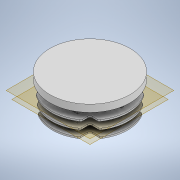
# Autodesk Inventor part: Plug
Saved by Autodesk Inventor 2020.2 (Build 242310000, 310)
## iProperties
Created: 2019-12-23
Part Number: Plug
Material: Générique
Document SubType Name: Modeling
Designer: damien
Density: 1 g/cm^3
Appearance: Par défaut
Author: damien
Autodesk Inventor part; units mm, degrees
ref_plane "YZ Plane" through (0, 0, 0) normal (1, 0, 0) x (0, 1, 0)
ref_plane "XZ Plane" through (0, 0, 0) normal (0, 1, 0) x (-1, 0, 0)
ref_plane "XY Plane" through (0, 0, 0) normal (0, 0, 1) x (1, 0, 0)
sketch "Esquisse1" plane through (0, 0, 0) normal (0, 1, 0) x (-1, 0, 0)
  line L0 (7.6, 13.55) -> (-7.6, 13.55)
  line L1 (-7.6, 13.55) -> (-7.6, 12.25)
  line L2 (-7.6, 12.25) -> (-0.65, 12.25)
  line L3 (-0.65, 12.25) -> (-0.65, 0.65)
  line L4 (-0.65, 0.65) -> (-15.5, 0.65)
  line L5 (-15.5, 0.65) -> (-15.5, -0.65)
  line L6 (-15.5, -0.65) -> (-0.65, -0.65)
  line L7 (-0.65, -0.65) -> (-0.65, -12.25)
  line L8 (-0.65, -12.25) -> (-7.6, -12.25)
  line L9 (-7.6, -12.25) -> (-7.6, -13.55)
  line L10 (-7.6, -13.55) -> (7.6, -13.55)
  line L11 (7.6, -13.55) -> (7.6, -12.25)
  line L12 (7.6, -12.25) -> (0.65, -12.25)
  line L13 (0.65, -12.25) -> (0.65, -0.65)
  line L14 (0.65, -0.65) -> (15.5, -0.65)
  line L15 (15.5, -0.65) -> (15.5, 0.65)
  line L16 (15.5, 0.65) -> (0.65, 0.65)
  line L17 (0.65, 0.65) -> (0.65, 12.25)
  line L18 (0.65, 12.25) -> (7.6, 12.25)
  line L19 (7.6, 12.25) -> (7.6, 13.55)
  line L20 (-0.65, 0.65) -> (0.65, -0.65) construction
  line L21 (0.65, 0.65) -> (-0.65, -0.65) construction
  point P0 (0, 0)
  point P1 (0, 0)
  dimension "d0" = 15.2
  dimension "d1" = 27.1
  dimension "d2" = 1.3
  dimension "d4" = 31
  dimension "d7" = 1.3
  constraints: 44 end point, 12 perpendicular, 11 point on line, 6 equal length, 2 horizontal, 1 coincident, 1 collinear, 1 midpoint, 1 parallel
  measures "d0" distance of L0.start L0.end
  measures "d1" distance between parallel lines of L10 L0
  measures "d2" distance of L18.end L0.start
  measures "d4" distance between parallel lines of L5 L15
  measures "d7" distance between parallel lines of L3 L17
extrude "Extrusion1" add sketch "Esquisse1" along normal blind 15.35
sketch "Esquisse2" plane through (0, 15.35, 0) normal (0, 1, 0) x (1, 0, 0)
  line L0 (0, -19.15) -> (0, -13.55) construction
  line L1 (-7.6, -13.55) -> (7.6, -13.55) construction
  circle A0 centre (0, 0) radius 19.15
  dimension "d8" = 5.6
  constraints: 2 end point, 1 coincident, 1 midpoint, 1 vertical, 1 vertical alignment, 2 other
  measures "d8" distance of L0.start L0.end
extrude "Extrusion2" add sketch "Esquisse2" against normal blind 3.4
sketch "Esquisse5" plane through (0, 0, 0) normal (0, -1, 0) x (1, 0, 0)
  circle A0 centre (0, 0) radius 14 construction
  line L0 (-14.4844, 9.8995) -> (-10.8995, 9.8995)
  line L1 (-9.8995, 14.4844) -> (-9.8995, 10.8995)
  arc A1 (-10.8995, 9.8995) -> (-9.8995, 10.8995) centre (-10.8995, 10.8995) ccw
  line L2 (0, 18) -> (0, -17.3614) construction
  line L3 (18, 0) -> (-18, 0) construction
  line L4 (-15.0333, -9.8995) -> (-10.8995, -9.8995)
  line L5 (-9.8995, -14.4844) -> (-9.8995, -10.8995)
  arc A2 (-9.8995, -10.8995) -> (-10.8995, -9.8995) centre (-10.8995, -10.8995) ccw
  line L6 (14.4844, 9.8995) -> (10.8995, 9.8995)
  line L7 (9.8995, 14.4844) -> (9.8995, 10.8995)
  arc A3 (9.8995, 10.8995) -> (10.8995, 9.8995) centre (10.8995, 10.8995) ccw
  line L8 (9.8995, -14.4844) -> (9.8995, -10.8995)
  line L9 (14.4844, -9.8995) -> (10.8995, -9.8995)
  arc A4 (10.8995, -9.8995) -> (9.8995, -10.8995) centre (10.8995, -10.8995) ccw
  arc A5 (-15.3365, 9.423) -> (-15.0333, -9.8995) centre (0, 0) ccw
  arc A6 (9.423, 15.3365) -> (-9.423, 15.3365) centre (0, 0) ccw
  arc A7 (-9.423, -15.3365) -> (9.423, -15.3365) centre (0, 0) ccw
  arc A8 (15.3365, -9.423) -> (15.3365, 9.423) centre (0, 0) ccw
  arc A9 (9.423, -15.3365) -> (9.8995, -14.4844) centre (8.8995, -14.4844) ccw
  arc A10 (-9.8995, -14.4844) -> (-9.423, -15.3365) centre (-8.8995, -14.4844) ccw
  arc A11 (14.4844, -9.8995) -> (15.3365, -9.423) centre (14.4844, -8.8995) ccw
  arc A12 (15.3365, 9.423) -> (14.4844, 9.8995) centre (14.4844, 8.8995) ccw
  arc A13 (9.8995, 14.4844) -> (9.423, 15.3365) centre (8.8995, 14.4844) ccw
  arc A14 (-9.423, 15.3365) -> (-9.8995, 14.4844) centre (-8.8995, 14.4844) ccw
  arc A15 (-14.4844, 9.8995) -> (-15.3365, 9.423) centre (-14.4844, 8.8995) ccw
  point P0 (-15.0333, 9.8995)
  point P1 (-9.8995, 9.8995)
  point P2 (-9.8995, 15.0333)
  point P3 (-9.8995, -15.0333)
  point P4 (15.0333, 9.8995)
  point P5 (9.8995, 15.0333)
  point P6 (9.8995, -15.0333)
  point P7 (15.0333, -9.8995)
  dimension "d16" = 28
  dimension "d18" = 1
  dimension "d19" = 18
  dimension "d20" = 18
  dimension "d28" = 1
  constraints: 40 point on circle, 20 end point, 17 symmetric about line, 16 tangent, 15 centre point, 10 point on line, 6 equal radius, 2 coincident, 2 horizontal, 2 perpendicular, 1 midpoint, 1 vertical, 6 other
  measures "d18" radius of A1
  measures "d19" radius of A5
  measures "d20" radius of A7
  measures "d28" radius of A9
extrude "Extrusion4" add sketch "Esquisse5" against normal blind 0.75
ref_plane "Plan de construction2" through (0, 3.75, 0) normal (0, 1, 0) x (1, 0, 0)
sketch "Esquisse6" plane through (0, 3.75, 0) normal (0, 1, 0) x (1, 0, 0)
  circle A0 centre (0, 0) radius 19.15 projected
  line L0 (14.9971, 10.3995) -> (11.3995, 10.3995)
  line L1 (10.3995, 11.3995) -> (10.3995, 14.9971)
  arc A1 (10.3995, 11.3995) -> (11.3995, 10.3995) centre (11.3995, 11.3995) ccw
  line L2 (-10.3995, -14.9971) -> (-10.3995, -11.3995)
  line L3 (-11.3995, -10.3995) -> (-14.9971, -10.3995)
  arc A2 (-10.3995, -11.3995) -> (-11.3995, -10.3995) centre (-11.3995, -11.3995) ccw
  line L4 (10.8995, 9.8995) -> (14.4844, 9.8995) projected
  line L5 (-9.8995, -14.4844) -> (-9.8995, -10.8995) projected
  arc A3 (-9.423, -15.3365) -> (9.423, -15.3365) centre (0, 0) ccw projected
  line L6 (0, -18) -> (0, 18) construction
  arc A4 (9.423, 15.3365) -> (-9.423, 15.3365) centre (0, 0) ccw projected
  line L7 (-14.9971, 10.3995) -> (-11.3995, 10.3995)
  line L8 (-10.3995, 11.3995) -> (-10.3995, 14.9971)
  arc A5 (-11.3995, 10.3995) -> (-10.3995, 11.3995) centre (-11.3995, 11.3995) ccw
  line L9 (10.3995, -14.9971) -> (10.3995, -11.3995)
  line L10 (11.3995, -10.3995) -> (14.9971, -10.3995)
  arc A6 (11.3995, -10.3995) -> (10.3995, -11.3995) centre (11.3995, -11.3995) ccw
  arc A7 (14.9971, -10.3995) -> (14.9971, 10.3995) centre (0, 0) ccw
  arc A8 (10.3995, 14.9971) -> (-10.3995, 14.9971) centre (0, 0) ccw
  arc A9 (-14.9971, 10.3995) -> (-14.9971, -10.3995) centre (0, 0) ccw
  arc A10 (-10.3995, -14.9971) -> (10.3995, -14.9971) centre (0, 0) ccw
  dimension "d25" = 1
  dimension "d26" = 1
  dimension "d29" = 0.5
  dimension "d30" = 0.5
  dimension "d31" = 18.25
  dimension "d32" = 18.25
  dimension "d33" = 18.25
  constraints: 18 end point, 18 point on circle, 10 symmetric about line, 8 centre point, 4 perpendicular, 4 tangent, 2 vertical, 1 coincident, 1 horizontal, 1 midpoint, 2 other
  measures "d25" radius of A1
  measures "d26" radius of A2
  measures "d29" distance between parallel lines of L4 L0
  measures "d30" distance between parallel lines of L5 L2
  measures "d31" radius of A7
  measures "d32" radius of A8
  measures "d33" radius of A10
extrude "Extrusion5" add sketch "Esquisse6" along normal blind 0.75 contours A7 L10 A6 L9 A10 L2 A2 L3 A9 L7 A5 L8 A8 L1 A1 L0
ref_plane "Plan de construction3" through (0, 7.5, 0) normal (0, 1, 0) x (1, 0, 0)
sketch "Esquisse7" plane through (0, 7.5, 0) normal (0, 1, 0) x (1, 0, 0)
  line L0 (14.9483, 10.8995) -> (11.8995, 10.8995)
  line L1 (10.8995, 11.8995) -> (10.8995, 14.9483)
  arc A0 (10.8995, 11.8995) -> (11.8995, 10.8995) centre (11.8995, 11.8995) ccw
  line L2 (14.9971, 10.3995) -> (11.3995, 10.3995) projected
  line L3 (-10.8995, 14.9483) -> (-10.8995, 11.8995)
  line L4 (-11.8995, 10.8995) -> (-14.9483, 10.8995)
  arc A1 (-11.8995, 10.8995) -> (-10.8995, 11.8995) centre (-11.8995, 11.8995) ccw
  line L5 (14.9483, -10.8995) -> (11.8995, -10.8995)
  line L6 (10.8995, -11.8995) -> (10.8995, -14.9483)
  arc A2 (11.8995, -10.8995) -> (10.8995, -11.8995) centre (11.8995, -11.8995) ccw
  line L7 (-10.8995, -14.9483) -> (-10.8995, -11.8995)
  line L8 (-11.8995, -10.8995) -> (-14.9483, -10.8995)
  arc A3 (-10.8995, -11.8995) -> (-11.8995, -10.8995) centre (-11.8995, -11.8995) ccw
  arc A4 (10.8995, 14.9483) -> (-10.8995, 14.9483) centre (0, 0) ccw
  arc A5 (14.9483, -10.8995) -> (14.9483, 10.8995) centre (0, 0) ccw
  arc A6 (-14.9483, 10.8995) -> (-14.9483, -10.8995) centre (0, 0) ccw
  arc A7 (-10.8995, -14.9483) -> (10.8995, -14.9483) centre (0, 0) ccw
  dimension "d39" = 1
  dimension "d40" = 0.5
  dimension "d41" = 1
  dimension "d42" = 1
  dimension "d43" = 1
  dimension "d44" = 18.5
  dimension "d45" = 18.5
  dimension "d46" = 18.5
  dimension "d47" = 18.5
  constraints: 16 end point, 16 point on circle, 8 centre point, 8 tangent, 4 equal length, 4 perpendicular, 3 collinear, 2 horizontal, 2 vertical, 1 coincident
  measures "d39" radius of A0
  measures "d40" distance between parallel lines of L2 L0
  measures "d41" radius of A1
  measures "d42" radius of A2
  measures "d43" radius of A3
  measures "d44" radius of A5
  measures "d45" radius of A4
  measures "d46" radius of A6
  measures "d47" radius of A7
extrude "Extrusion6" add sketch "Esquisse7" along normal blind 0.75
fillet "Congé1" radius 1 16 edges at (14.9483, 7.875, -10.8995) (14.9971, 4.125, -10.3995) (10.3995, 4.125, -14.9971) (10.8995, 7.875, -14.9483) (14.9483, 7.875, 10.8995) (14.9971, 4.125, 10.3995) (10.8995, 7.875, 14.9483) (10.3995, 4.125, 14.9971) (-10.8995, 7.875, 14.9483) (-10.3995, 4.125, 14.9971) (-14.9483, 7.875, 10.8995) (-14.9971, 4.125, 10.3995) (-14.9483, 7.875, -10.8995) (-14.9971, 4.125, -10.3995) (-10.8995, 7.875, -14.9483) (-10.3995, 4.125, -14.9971)
fillet "Congé2" radius 1 1 edges at (-15.0333, 0.375, -9.8995)
